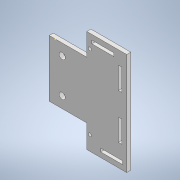
# Autodesk Inventor part: pcbek
Saved by Autodesk Inventor 2022 (Build 260153000, 153)
## iProperties
Created: 2023-01-27
Part Number: pcbek
Material: Generic
Document SubType Name: Modeling
Designer: Kamil
Density: 1 g/cm^3
Appearance: Default
Author: Kamil
Autodesk Inventor part; units mm, degrees
ref_plane "YZ Plane" through (0, 0, 0) normal (1, 0, 0) x (0, 1, 0)
ref_plane "XZ Plane" through (0, 0, 0) normal (0, 1, 0) x (-1, 0, 0)
ref_plane "XY Plane" through (0, 0, 0) normal (0, 0, 1) x (1, 0, 0)
sketch "Sketch1" plane through (0, 0, 0) normal (0, 0, 1) x (1, 0, 0)
  circle A0 centre (3.2816, -5.4552) radius 1.5 projected
  line L0 (4.45, -12.0667) -> (7.65, -10.2192) projected
  line L1 (7.65, -10.2192) -> (10.85, -12.0667) projected
  line L2 (10.85, -12.0667) -> (10.85, -15.7617) projected
  line L3 (10.85, -15.7617) -> (7.65, -17.6093) projected
  line L4 (7.65, -17.6093) -> (4.45, -15.7617) projected
  line L5 (4.45, -15.7617) -> (4.45, -12.0667) projected
  circle A1 centre (3.2816, -22.3733) radius 1.5 projected
  line L6 (15.3, -27.8284) -> (15.3, 0) projected
  line L7 (0, 0) -> (15.3, 0) projected
  line L8 (0, -27.8284) -> (0, 0) projected
  line L9 (0, -27.8284) -> (15.3, -27.8284) projected
  line L10 (28.3, 5.8858) -> (15.3, 5.8858) projected
  line L11 (15.3, 5.8858) -> (15.3, -34.1142) projected
  line L12 (28.3, -34.1142) -> (15.3, -34.1142) projected
  line L13 (28.3, 5.8858) -> (28.3, -34.1142) projected
  line L14 (38.8108, -39.1142) -> (38.8108, 10.8858) projected
  line L15 (38.8108, 10.8858) -> (15.3, 10.8858) projected
  line L16 (15.3, -2.6142) -> (15.3, 10.8858) projected
  line L17 (15.3, -2.6142) -> (38.3, -2.6142) projected
  line L18 (38.3, -12.6142) -> (38.3, -2.6142) projected
  line L19 (38.3, -12.6142) -> (7.65, -12.6142) projected
  arc A2 (7.65, -15.6142) -> (7.65, -12.6142) centre (7.65, -14.1142) ccw projected
  line L20 (7.65, -15.6142) -> (38.3, -15.6142) projected
  line L21 (38.3, -25.6142) -> (38.3, -15.6142) projected
  line L22 (38.3, -25.6142) -> (15.3, -25.6142) projected
  line L23 (15.3, -39.1142) -> (15.3, -25.6142) projected
  line L24 (38.8108, -39.1142) -> (15.3, -39.1142) projected
  line L25 (-7.04, -39.1142) -> (14.96, -39.1142) projected
  line L26 (-7.04, -39.1142) -> (38.8108, -39.1142)
  line L27 (38.8108, -39.1142) -> (38.8108, 10.8858)
  line L28 (38.8108, 10.8858) -> (-7.04, 10.8858)
  line L29 (-7.04, 10.8858) -> (-7.04, -39.1142)
  line L30 (-5.04, -27.8284) -> (13.16, -27.8284) projected
  line L31 (13.16, 0) -> (-5.04, 0) projected
  line L32 (-3.04, -35.1142) -> (34.8108, -35.1142)
  line L33 (34.8108, -35.1142) -> (34.8108, 6.8858)
  line L34 (34.8108, 6.8858) -> (-3.04, 6.8858)
  line L35 (-3.04, 6.8858) -> (-3.04, -35.1142)
  line L36 (34.8108, -35.1142) -> (15.3, -35.1142)
  line L37 (15.3, -35.1142) -> (15.3, -39.1142)
  line L38 (15.3, -39.1142) -> (34.8108, -39.1142)
  line L39 (34.8108, -39.1142) -> (34.8108, -35.1142)
  line L40 (15.3, 6.8858) -> (34.8108, 6.8858)
  line L41 (34.8108, 6.8858) -> (34.8108, 10.8858)
  line L42 (34.8108, 10.8858) -> (15.3, 10.8858)
  line L43 (15.3, 10.8858) -> (15.3, 6.8858)
  point P0 (-3.04, 0)
  point P1 (-3.04, -27.8284)
  dimension "d0" = 4
  constraints: 32 end point, 8 parallel, 4 perpendicular, 4 point on line, 3 horizontal, 3 other
  measures "d0" distance between parallel lines of L29 L35
extrude "Extrusion1" add sketch "Sketch1" along normal blind 2 contours L5 L4 L3 L2 L20 L6 L9 L8 L7 L19 L1 L0 | L0 L1 L2 L19 A2 L20 L3 L4 L5 | L19 L6 L20 L2 | L2 L20 A2 L19 | L19 L13 L20 L6 | L6 L17 L13 L19 | L20 L13 L22 L6 | L6 L11 L10 L13 L17 | L19 L33 L20 L13 | L13 L17 L33 L19 | L22 L13 L12 L11 L6 | L20 L33 L22 L13 | L13 L10 L16 L34 L33 L17 | L33 L17 L18 L19 | L19 L18 L17 L33 L41 L15 L14 L24 L39 L22 L21 L20 | L22 L33 L32 L23 L12 L13 | L20 L21 L22 L33 | L8 L30 L35 L31 | L16 L15 L41 L34 | L32 L39 L24 L23
sketch "Sketch2" plane through (0, 0, 2) normal (0, 0, 1) x (1, 0, 0)
  line L0 (15.3, 0) -> (-3.04, 0) projected
  line L1 (-3.04, 0) -> (-3.04, -27.8284) projected
  line L2 (-3.04, -27.8284) -> (15.3, -27.8284) projected
  line L3 (15.3, -27.8284) -> (15.3, -39.1142) projected
  line L4 (15.3, -39.1142) -> (38.8108, -39.1142) projected
  line L5 (38.8108, -39.1142) -> (38.8108, 10.8858) projected
  line L6 (38.8108, 10.8858) -> (15.3, 10.8858) projected
  line L7 (15.3, 10.8858) -> (15.3, 0) projected
  circle A0 centre (3.2816, -22.3733) radius 1.5 projected
  circle A1 centre (3.2816, -5.4552) radius 1.5 projected
  line L8 (15.3, -39.1142) -> (38.8108, -39.1142) projected
  line L9 (38.8108, 10.8858) -> (34.8108, 10.8858)
  line L10 (34.8108, 10.8858) -> (34.8108, -39.1142)
  line L11 (34.8108, -39.1142) -> (38.8108, -39.1142)
  line L12 (38.8108, -39.1142) -> (38.8108, 10.8858)
  point P0 (0, 0)
  dimension "d3" = 4
  constraints: 8 end point, 2 parallel, 1 horizontal, 1 perpendicular, 1 point on line
  measures "d3" distance of L11.end L10.end
extrude "Extrusion2" cut sketch "Sketch2" against normal blind 2 contours L6 L5 L4 L10
sketch "Sketch3" plane through (0, 0, 2) normal (0, 0, 1) x (1, 0, 0)
  point P0 (0, 0)
sketch "Sketch4" plane through (0, 0, 2) normal (0, 0, 1) x (1, 0, 0)
  circle A0 centre (16.8, -32.0784) radius 0.75 projected
  circle A1 centre (16.8, 4.25) radius 0.75 projected
  point P0 (0, 0)
extrude "Extrusion3" cut sketch "Sketch4" against normal through all
sketch "Sketch5" plane through (0, 0, 2) normal (0, 0, 1) x (1, 0, 0)
  circle A0 centre (16.8, 4.25) radius 0.75 projected
  circle A1 centre (16.8, -32.0784) radius 0.75 projected
  line L0 (34.8108, -39.1142) -> (34.8108, 10.8858) projected
  line L1 (34.8108, 10.8858) -> (15.3, 10.8858) projected
  line L2 (15.3, 10.8858) -> (15.3, 0) projected
  line L3 (15.3, 0) -> (-3.04, 0) projected
  line L4 (-3.04, 0) -> (-3.04, -27.8284) projected
  line L5 (-3.04, -27.8284) -> (15.3, -27.8284) projected
  line L6 (15.3, -27.8284) -> (15.3, -39.1142) projected
  line L7 (15.3, -39.1142) -> (34.8108, -39.1142) projected
  circle A2 centre (3.2816, -22.3733) radius 1.5 projected
  circle A3 centre (3.2816, -5.4552) radius 1.5 projected
  line L8 (22.1108, -36.7142) -> (32.8108, -36.7142) projected
  line L9 (22.1108, -36.7142) -> (22.1108, -35.1142) projected
  line L10 (32.8108, -35.1142) -> (22.1108, -35.1142) projected
  line L11 (32.8108, -36.7142) -> (32.8108, -35.1142) projected
  line L12 (32.4108, -28.3142) -> (32.4108, -17.6142) projected
  line L13 (32.4108, -28.3142) -> (30.8108, -28.3142) projected
  line L14 (30.8108, -17.6142) -> (30.8108, -28.3142) projected
  line L15 (32.4108, -17.6142) -> (30.8108, -17.6142) projected
  line L16 (32.4108, -6.3142) -> (32.4108, 4.3858) projected
  line L17 (32.4108, -6.3142) -> (30.8108, -6.3142) projected
  line L18 (30.8108, 4.3858) -> (30.8108, -6.3142) projected
  line L19 (32.4108, 4.3858) -> (30.8108, 4.3858) projected
  line L20 (32.8108, 8.4858) -> (22.1108, 8.4858) projected
  line L21 (32.8108, 8.4858) -> (32.8108, 6.8858) projected
  line L22 (22.1108, 6.8858) -> (32.8108, 6.8858) projected
  line L23 (22.1108, 8.4858) -> (22.1108, 6.8858) projected
  point P0 (0, 0)
extrude "Extrusion4" cut sketch "Sketch5" against normal through all contours L9 L10 L11 L8 | L13 L14 L15 L12 | L17 L18 L19 L16 | L21 L22 L23 L20
sketch "Sketch6" plane through (0, 0, 2) normal (0, 0, 1) x (1, 0, 0)
  line L0 (30.8108, -28.3142) -> (30.8108, -17.6142) projected
  line L1 (30.8108, -17.6142) -> (32.4108, -17.6142) projected
  line L2 (32.4108, -17.6142) -> (32.4108, -28.3142) projected
  line L3 (32.4108, -28.3142) -> (30.8108, -28.3142) projected
  line L4 (30.8108, -6.3142) -> (30.8108, 4.3858) projected
  line L5 (30.8108, 4.3858) -> (32.4108, 4.3858) projected
  line L6 (32.4108, 4.3858) -> (32.4108, -6.3142) projected
  line L7 (32.4108, -6.3142) -> (30.8108, -6.3142) projected
  line L8 (22.1108, -35.1142) -> (32.8108, -35.1142) projected
  line L9 (32.8108, -35.1142) -> (32.8108, -36.7142) projected
  line L10 (32.8108, -36.7142) -> (22.1108, -36.7142) projected
  line L11 (22.1108, -36.7142) -> (22.1108, -35.1142) projected
  line L12 (32.8108, 6.8858) -> (22.1108, 6.8858) projected
  line L13 (22.1108, 6.8858) -> (22.1108, 8.4858) projected
  line L14 (22.1108, 8.4858) -> (32.8108, 8.4858) projected
  line L15 (32.8108, 8.4858) -> (32.8108, 6.8858) projected
  circle A0 centre (16.8, 4.25) radius 0.75 projected
  circle A1 centre (16.8, -32.0784) radius 0.75 projected
  line L16 (34.8108, -39.1142) -> (34.8108, 10.8858) projected
  line L17 (34.8108, 10.8858) -> (15.3, 10.8858) projected
  line L18 (15.3, 10.8858) -> (15.3, 0) projected
  line L19 (15.3, 0) -> (-3.04, 0) projected
  line L20 (-3.04, 0) -> (-3.04, -27.8284) projected
  line L21 (-3.04, -27.8284) -> (15.3, -27.8284) projected
  line L22 (15.3, -27.8284) -> (15.3, -39.1142) projected
  line L23 (15.3, -39.1142) -> (34.8108, -39.1142) projected
  circle A2 centre (3.2816, -22.3733) radius 1.5 projected
  circle A3 centre (3.2816, -5.4552) radius 1.5 projected
  line L24 (34.8108, 10.8858) -> (15.3, 10.8858) projected
  line L25 (15.3, 10.8858) -> (15.3, 0) projected
  line L26 (34.8108, 10.8858) -> (15.3, 10.8858)
  line L27 (15.3, 10.8858) -> (15.3, 10.0858)
  line L28 (15.3, 10.0858) -> (34.8108, 10.0858)
  line L29 (34.8108, 10.0858) -> (34.8108, 10.8858)
  line L30 (15.3, -27.8284) -> (15.3, -39.1142) projected
  line L31 (34.8108, 10.8858) -> (34.8108, -39.1142) projected
  line L32 (15.3, -39.1142) -> (34.8108, -39.1142)
  line L33 (34.8108, -39.1142) -> (34.8108, -38.3142)
  line L34 (34.8108, -38.3142) -> (15.3, -38.3142)
  line L35 (15.3, -38.3142) -> (15.3, -39.1142)
  point P0 (0, 0)
  dimension "d10" = 0.8
  dimension "d11" = 0.8
  constraints: 16 end point, 4 parallel, 2 horizontal, 2 perpendicular, 2 point on line
  measures "d10" distance of L27.end L26.end
  measures "d11" distance of L33.end L32.end
extrude "Extrusion5" cut sketch "Sketch6" against normal through all contours L23 L22 L34 L16 | L28 L18 L17 L16
sketch "Sketch7" plane through (0, 0, 2) normal (0, 0, 1) x (1, 0, 0)
  line L0 (34.8108, 10.0858) -> (15.3, 10.0858) projected
  line L1 (15.3, 10.0858) -> (15.3, 0) projected
  line L2 (15.3, 0) -> (-3.04, 0) projected
  line L3 (-3.04, 0) -> (-3.04, -27.8284) projected
  line L4 (-3.04, -27.8284) -> (15.3, -27.8284) projected
  line L5 (15.3, -27.8284) -> (15.3, -38.3142) projected
  line L6 (15.3, -38.3142) -> (34.8108, -38.3142) projected
  line L7 (34.8108, -38.3142) -> (34.8108, 10.0858) projected
  line L8 (30.8108, -28.3142) -> (30.8108, -17.6142) projected
  line L9 (30.8108, -17.6142) -> (32.4108, -17.6142) projected
  line L10 (32.4108, -17.6142) -> (32.4108, -28.3142) projected
  line L11 (32.4108, -28.3142) -> (30.8108, -28.3142) projected
  line L12 (30.8108, -6.3142) -> (30.8108, 4.3858) projected
  line L13 (30.8108, 4.3858) -> (32.4108, 4.3858) projected
  line L14 (32.4108, 4.3858) -> (32.4108, -6.3142) projected
  line L15 (32.4108, -6.3142) -> (30.8108, -6.3142) projected
  line L16 (22.1108, -35.1142) -> (32.8108, -35.1142) projected
  line L17 (32.8108, -35.1142) -> (32.8108, -36.7142) projected
  line L18 (32.8108, -36.7142) -> (22.1108, -36.7142) projected
  line L19 (22.1108, -36.7142) -> (22.1108, -35.1142) projected
  line L20 (32.8108, 6.8858) -> (22.1108, 6.8858) projected
  line L21 (22.1108, 6.8858) -> (22.1108, 8.4858) projected
  line L22 (22.1108, 8.4858) -> (32.8108, 8.4858) projected
  line L23 (32.8108, 8.4858) -> (32.8108, 6.8858) projected
  circle A0 centre (16.8, 4.25) radius 0.75 projected
  circle A1 centre (16.8, -32.0784) radius 0.75 projected
  circle A2 centre (3.2816, -22.3733) radius 1.5 projected
  circle A3 centre (3.2816, -5.4552) radius 1.5 projected
  line L24 (38.8108, 10.8858) -> (15.3, 10.8858) projected
  line L25 (38.8108, -39.1142) -> (15.3, -39.1142) projected
  line L26 (15.3, 10.0858) -> (34.8108, 10.0858) projected
  line L27 (15.3, 10.8858) -> (34.8108, 10.8858)
  line L28 (34.8108, 10.8858) -> (34.8108, 10.0858)
  line L29 (34.8108, 10.0858) -> (15.3, 10.0858)
  line L30 (15.3, 10.0858) -> (15.3, 10.8858)
  line L31 (34.8108, -38.3142) -> (15.3, -38.3142) projected
  line L32 (34.8108, -38.3142) -> (15.3, -38.3142)
  line L33 (15.3, -38.3142) -> (15.3, -39.1142)
  line L34 (15.3, -39.1142) -> (34.8108, -39.1142)
  line L35 (34.8108, -39.1142) -> (34.8108, -38.3142)
  point P0 (0, 0)
  constraints: 16 end point, 4 parallel, 2 horizontal, 2 perpendicular
extrude "Extrusion6" add sketch "Sketch7" against normal up to surface (2 mm away) contours L0 L30 L24 L28 | L35 L25 L33 L6
sketch "Sketch8" plane through (0, 0, 2) normal (0, 0, 1) x (1, 0, 0)
  line L0 (15.3, 10.8858) -> (15.3, 0) projected
  line L1 (15.3, 0) -> (-3.04, 0) projected
  line L2 (-3.04, 0) -> (-3.04, -27.8284) projected
  line L3 (-3.04, -27.8284) -> (15.3, -27.8284) projected
  line L4 (15.3, -27.8284) -> (15.3, -39.1142) projected
  line L5 (15.3, -39.1142) -> (34.8108, -39.1142) projected
  line L6 (34.8108, -39.1142) -> (34.8108, 10.8858) projected
  line L7 (34.8108, 10.8858) -> (15.3, 10.8858) projected
  line L8 (30.8108, -28.3142) -> (30.8108, -17.6142) projected
  line L9 (30.8108, -17.6142) -> (32.4108, -17.6142) projected
  line L10 (32.4108, -17.6142) -> (32.4108, -28.3142) projected
  line L11 (32.4108, -28.3142) -> (30.8108, -28.3142) projected
  line L12 (30.8108, -6.3142) -> (30.8108, 4.3858) projected
  line L13 (30.8108, 4.3858) -> (32.4108, 4.3858) projected
  line L14 (32.4108, 4.3858) -> (32.4108, -6.3142) projected
  line L15 (32.4108, -6.3142) -> (30.8108, -6.3142) projected
  line L16 (22.1108, -35.1142) -> (32.8108, -35.1142) projected
  line L17 (32.8108, -35.1142) -> (32.8108, -36.7142) projected
  line L18 (32.8108, -36.7142) -> (22.1108, -36.7142) projected
  line L19 (22.1108, -36.7142) -> (22.1108, -35.1142) projected
  line L20 (32.8108, 6.8858) -> (22.1108, 6.8858) projected
  line L21 (22.1108, 6.8858) -> (22.1108, 8.4858) projected
  line L22 (22.1108, 8.4858) -> (32.8108, 8.4858) projected
  line L23 (32.8108, 8.4858) -> (32.8108, 6.8858) projected
  circle A0 centre (16.8, 4.25) radius 0.75 projected
  circle A1 centre (16.8, -32.0784) radius 0.75 projected
  circle A2 centre (3.2816, -22.3733) radius 1.5 projected
  circle A3 centre (3.2816, -5.4552) radius 1.5 projected
  line L24 (28.5108, 8.4858) -> (17.8108, 8.4858) projected
  line L25 (28.5108, 8.4858) -> (28.5108, 6.8858) projected
  line L26 (17.8108, 6.8858) -> (28.5108, 6.8858) projected
  line L27 (17.8108, 8.4858) -> (17.8108, 6.8858) projected
  point P0 (0, 0)
extrude "Extrusion7" cut sketch "Sketch8" against normal blind 10 contours L26 L27 L24 L21
sketch "Sketch9" plane through (0, 0, 2) normal (0, 0, 1) x (1, 0, 0)
  circle A0 centre (3.2816, -5.4552) radius 1.5 projected
  circle A1 centre (3.2816, -22.3733) radius 1.5 projected
  circle A2 centre (16.8, -32.0784) radius 0.75 projected
  circle A3 centre (16.8, 4.25) radius 0.75 projected
  line L0 (32.8108, 6.8858) -> (17.8108, 6.8858) projected
  line L1 (17.8108, 6.8858) -> (17.8108, 8.4858) projected
  line L2 (17.8108, 8.4858) -> (32.8108, 8.4858) projected
  line L3 (32.8108, 8.4858) -> (32.8108, 6.8858) projected
  line L4 (22.1108, -35.1142) -> (32.8108, -35.1142) projected
  line L5 (32.8108, -35.1142) -> (32.8108, -36.7142) projected
  line L6 (32.8108, -36.7142) -> (22.1108, -36.7142) projected
  line L7 (22.1108, -36.7142) -> (22.1108, -35.1142) projected
  line L8 (30.8108, -6.3142) -> (30.8108, 4.3858) projected
  line L9 (30.8108, 4.3858) -> (32.4108, 4.3858) projected
  line L10 (32.4108, 4.3858) -> (32.4108, -6.3142) projected
  line L11 (32.4108, -6.3142) -> (30.8108, -6.3142) projected
  line L12 (30.8108, -28.3142) -> (30.8108, -17.6142) projected
  line L13 (30.8108, -17.6142) -> (32.4108, -17.6142) projected
  line L14 (32.4108, -17.6142) -> (32.4108, -28.3142) projected
  line L15 (32.4108, -28.3142) -> (30.8108, -28.3142) projected
  line L16 (15.3, 10.8858) -> (15.3, 0) projected
  line L17 (15.3, 0) -> (-3.04, 0) projected
  line L18 (-3.04, 0) -> (-3.04, -27.8284) projected
  line L19 (-3.04, -27.8284) -> (15.3, -27.8284) projected
  line L20 (15.3, -27.8284) -> (15.3, -39.1142) projected
  line L21 (15.3, -39.1142) -> (34.8108, -39.1142) projected
  line L22 (34.8108, -39.1142) -> (34.8108, 10.8858) projected
  line L23 (34.8108, 10.8858) -> (15.3, 10.8858) projected
  line L24 (28.5108, 8.4858) -> (28.5108, 6.8858) projected
  point P0 (0, 0)
extrude "Extrusion8" add sketch "Sketch9" against normal up to surface (2 mm away) contours L0 L24 L2 L3
body "Solid1"
